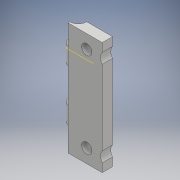
# Autodesk Inventor part: k2_hinge1_bot
Saved by Autodesk Inventor 2017 (Build 210142000, 142)
## iProperties
Created: 2017-02-14
Part Number: k2_hinge1_bot
Material: Generic
Document SubType Name: Modeling
Designer: herman
Density: 1 g/cm^3
Appearance: Default
Author: herman
Autodesk Inventor part; units mm, degrees
ref_plane "YZ Plane" through (0, 0, 0) normal (1, 0, 0) x (0, 1, 0)
ref_plane "XZ Plane" through (0, 0, 0) normal (0, 1, 0) x (-1, 0, 0)
ref_plane "XY Plane" through (0, 0, 0) normal (0, 0, 1) x (1, 0, 0)
sketch "Sketch2" plane through (0, 0, 0) normal (0, 1, 0) x (-1, 0, 0)
  line L0 (8.7236, 13.4517) -> (-1.2764, 13.4517)
  line L1 (-1.2764, 13.4517) -> (-1.2764, -3.0483)
  line L2 (-1.2764, -3.0483) -> (8.7236, -3.0483)
  line L3 (8.7236, -3.0483) -> (8.7236, 13.4517)
  point P0 (0, 0)
  dimension "d2" = 10
  dimension "d3" = 16.5
  constraints: 8 end point, 2 parallel, 1 horizontal, 1 perpendicular
  measures "d2" distance of L2.end L1.end
  measures "d3" distance of L1.end L0.end
extrude "Extrusion1" add sketch "Sketch2" along normal blind 3
ref_plane "Work Plane1" through (-8.7236, 0, 6.9517) normal (0, 0, 1) x (1, 0, 0)
sketch "Sketch5" plane through (-8.7236, 0, 13.4517) normal (0, 0, 1) x (1, 0, 0)
  line L0 (0, 3) -> (10, 3) projected
  circle A0 centre (0, 3) radius 2.5
  point P0 (8.7236, 0)
  dimension "d13" = 5
  constraints: 1 centre point
  measures "d13" diameter of A0
extrude "Extrusion4" cut sketch "Sketch5" against normal up to next
sketch "Sketch6" plane through (-8.7236, 0, 6.9517) normal (0, 0, 1) x (1, 0, 0)
  circle A0 centre (0, 3) radius 2.5
  arc A1 (0, 0.5) -> (2.5, 3) centre (0, 3) ccw projected
  point P0 (8.7236, 0)
  dimension "d16" = 5
  constraints: 1 centre point, 1 coincident
  measures "d16" diameter of A0
extrude "Extrusion5" add sketch "Sketch6" against normal blind 5
sketch "Sketch7" plane through (-8.7236, 0, 6.9517) normal (0, 0, 1) x (1, 0, 0)
  arc A0 (0, 0.5) -> (2.5, 3) centre (0, 3) ccw projected
  arc A1 (2.5, 3) -> (0, 0.5) centre (0, 3) ccw projected
  circle A2 centre (0, 3) radius 1.5
  point P0 (8.7236, 0)
  dimension "d20" = 3
  constraints: 1 centre point, 1 coincident
  measures "d20" diameter of A2
extrude "Extrusion6" cut sketch "Sketch7" against normal up to next contours A2
sketch "Sketch9" plane through (0, 3, 0) normal (0, 1, 0) x (1, 0, 0)
  circle A0 centre (-3.2236, -9.4517) radius 1.5
  line L0 (1.2764, -13.4517) -> (1.2764, 3.0483) projected
  line L1 (-6.2236, -13.4517) -> (1.2764, -13.4517) projected
  point P0 (0, 0)
  dimension "d28" = 3
  dimension "d29" = 4.5
  dimension "d30" = 4
  constraints: 1 centre point
  measures "d28" diameter of A0
  measures "d29" distance from line of L0 A0.centre
  measures "d30" distance from line of A0.centre L1
extrude "Extrusion8" cut sketch "Sketch9" against normal up to next
mirror "Mirror2" about plane through (1.2764, 0, -3.0483) normal (0, 0, -1)
sketch "Sketch10" plane through (0, 3, 0) normal (0, 1, 0) x (1, 0, 0)
  circle A0 centre (3.2764, -9.4517) radius 2.5
  circle A1 centre (3.2764, 15.5483) radius 2.5
  line L0 (1.2764, -13.4517) -> (1.2764, 19.5483) projected
  point P0 (0, 0)
  dimension "d33" = 5
  dimension "d34" = 5
  dimension "d35" = 2
  dimension "d36" = 4
  dimension "d37" = 4
  dimension "d40" = 2
  constraints: 2 centre point
  measures "d33" diameter of A0
  measures "d34" diameter of A1
  measures "d35" distance from line of L0 A0.centre
  measures "d36" vertical distance of L0.start A0.centre
  measures "d37" vertical distance of L0.end A1.centre
  measures "d40" distance from line of L0 A1.centre
extrude "Extrusion9" cut sketch "Sketch10" against normal through all
equation "\"d34\" = d33"
equation "\"d37\" = d36"
equation "\"d40\" = d35"
body "Solid1"
